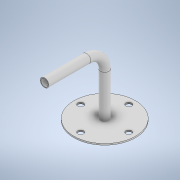
# Autodesk Inventor part: fractionating_column_cover
Saved by Autodesk Inventor 2020 (Build 240168000, 168)
## iProperties
Created: 2022-08-31
Part Number: fractionating_column_cover
Material: Generic
Document SubType Name: Modeling
Designer: Intuito_PC
Density: 1 g/cm^3
Appearance: Default
Author: Intuito_PC
Autodesk Inventor part; units mm, degrees
ref_plane "YZ Plane" through (0, 0, 0) normal (1, 0, 0) x (0, 1, 0)
ref_plane "XZ Plane" through (0, 0, 0) normal (0, 1, 0) x (-1, 0, 0)
sketch "Sketch1" plane through (0, 0, 0) normal (0, 1, 0) x (-1, 0, 0)
  circle A0 centre (0, 0) radius 43
  dimension "d0" = 86
  constraints: 1 centre point, 1 coincident
  measures "d0" diameter of A0
extrude "Extrusion1" add sketch "Sketch1" along normal blind 2
sketch "Sketch2" plane through (0, 2, 0) normal (0, 1, 0) x (1, 0, 0)
  circle A0 centre (-33.6296, 0) radius 4
  point P0 (0, 0)
  dimension "d3" = 8
  dimension "d4" = 33.6296
  constraints: 1 centre point
  measures "d3" diameter of A0
  measures "d4" distance of point (0, 0) A0.centre
extrude "Extrusion2" cut sketch "Sketch2" against normal blind 2
pattern_circular "Circular Pattern1" count 4 over 360 about axis through (0, 0, 0) along (0, 1, 0) of "Extrusion2"
sketch "Sketch3" plane through (0, 2, 0) normal (0, 1, 0) x (1, 0, 0)
  point P0 (0, 0)
sketch "Sketch4" plane through (0, 0, 0) normal (1, 0, 0) x (0, 1, 0)
  line L0 (0, 0) -> (62.0568, 0)
  line L1 (87.4568, 84.1442) -> (87.4568, 25.4)
  arc A0 (62.0568, 0) -> (87.4568, 25.4) centre (62.0568, 25.4) ccw
  point P0 (87.4568, 0)
  dimension "d18" = 25.4
  constraints: 4 end point, 2 point on circle, 2 point on line, 2 tangent, 1 centre point, 1 horizontal, 1 perpendicular
  measures "d18" radius of A0
ref_plane "Work Plane1" through (0, 2, 0) normal (0, 1, 0) x (-1, 0, 0)
sketch "Sketch5" plane through (0, 2, 0) normal (0, 1, 0) x (-1, 0, 0)
  circle A0 centre (0, 0) radius 5
  circle A1 centre (0, 0) radius 6
  dimension "d11" = 10
  dimension "d12" = 1
  constraints: 2 centre point, 1 coincident
  measures "d11" diameter of A0
  measures "d12" radial gap between concentric circles of A0 A1
sweep "Sweep1" add profiles "Sketch5" path "Sketch4" separate body contours A0 | A1
shell "Shell1" thickness 1 removed faces 1 at (0.2643, 86.4344, 84.1442) bodies 2
sketch "Sketch6" plane through (0, 0, 0) normal (0, -1, 0) x (1, 0, 0)
  circle A0 centre (0, 0) radius 6 projected
  circle A1 centre (0, 0) radius 5
  constraints: 1 centre point, 1 coincident
extrude "Extrusion3" cut sketch "Sketch6" against normal blind 41.275 contours A1 bodies 2
body "Solid1"
body "Solid3"
